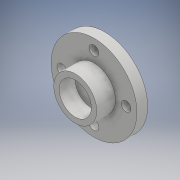
# Autodesk Inventor part: GWS_Micro2BBMG_hone_AS
Saved by Autodesk Inventor 2018.1 (Build 221171000, 171)
## iProperties
Created: 2017-10-25
Part Number: GWS_Micro2BBMG_hone_AS
Material: 一般
Document SubType Name: Modeling
Designer: sktom
Density: 1 g/cm^3
Appearance: 既定
Author: sktom
Autodesk Inventor part; units mm, degrees
ref_plane "YZ Plane" through (0, 0, 0) normal (1, 0, 0) x (0, 1, 0)
ref_plane "XZ Plane" through (0, 0, 0) normal (0, 1, 0) x (-1, 0, 0)
ref_plane "XY Plane" through (0, 0, 0) normal (0, 0, 1) x (1, 0, 0)
sketch "スケッチ1" plane through (0, 0, 0) normal (0, 0, 1) x (1, 0, 0)
  line L0 (0, 0) -> (-8, 0)
  line L1 (-8, 0) -> (-8, -2)
  line L2 (-8, -2) -> (-4, -2)
  line L3 (-4, -2) -> (-4, -5.5)
  line L4 (-4, -5.5) -> (-3, -5.5)
  line L5 (0, -2.5) -> (0, 0)
  line L6 (-3, -5.5) -> (-3, -2.5)
  line L7 (-3, -2.5) -> (0, -2.5)
  dimension "d0" = 2
  dimension "d1" = 3.5
  dimension "d2" = 8
  dimension "d4" = 4
  dimension "d5" = 0.5
  dimension "d6" = 3
  constraints: 16 end point, 6 perpendicular, 1 horizontal, 1 vertical
  measures "d0" distance of L0.end L1.end
  measures "d1" distance between parallel lines of L2 L4
  measures "d2" distance of L0.start L0.end
  measures "d4" distance between parallel lines of L5 L3
  measures "d5" distance between parallel lines of L2 L7
  measures "d6" distance between parallel lines of L5 L6
revolve "回転1" add sketch "スケッチ1" angle 360 about axis through (0, -2.5, 0) along (0, 1, 0)
sketch "スケッチ2" plane through (0, 0, 0) normal (0, 1, 0) x (1, 0, 0)
  circle A0 centre (0, 0) radius 0.9
  circle A1 centre (0, 0) radius 6 construction
  circle A2 centre (-6, 0) radius 0.9
  circle A3 centre (0, 6) radius 0.9
  circle A4 centre (6, 0) radius 0.9
  circle A5 centre (0, -6) radius 0.9
  dimension "d8" = 12
  dimension "d9" = 1.8
  constraints: 6 centre point, 4 equal radius, 4 point on circle, 2 coincident, 2 horizontal alignment, 2 vertical alignment
  measures "d8" diameter of A1
  measures "d9" diameter of A2
extrude "押し出し1" cut sketch "スケッチ2" against normal blind 10
